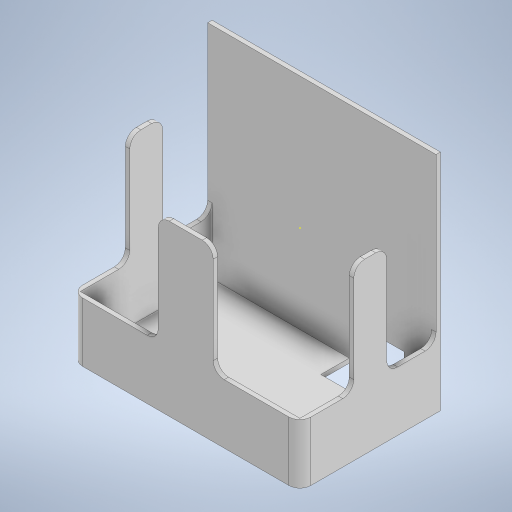
# Autodesk Inventor part: bag
Saved by Autodesk Inventor 2023 (Build 270158030, 158C)
## iProperties
Created: 2023-02-26
Part Number: bag
Material: Generic
Document SubType Name: Modeling
Designer: fatih
Density: 1 g/cm^3
Appearance: Default
Author: fatih
Autodesk Inventor part; units mm, degrees
ref_plane "YZ Plane" through (0, 0, 0) normal (1, 0, 0) x (0, 1, 0)
ref_plane "XZ Plane" through (0, 0, 0) normal (0, 1, 0) x (-1, 0, 0)
ref_plane "XY Plane" through (0, 0, 0) normal (0, 0, 1) x (1, 0, 0)
sketch "Sketch1" plane through (0, 0, 0) normal (0, 1, 0) x (-1, 0, 0)
  line L0 (0, 0) -> (0, -120)
  line L1 (0, 0) -> (200, 0)
  line L2 (200, 0) -> (200, -120)
  line L3 (200, -120) -> (0, -120)
  dimension "d0" = 120
  dimension "d1" = 200
  constraints: 8 end point, 2 perpendicular, 1 horizontal, 1 vertical
  measures "d0" distance of L0.start L0.end
  measures "d1" distance of L0.start L1.end
extrude "Extrusion1" add sketch "Sketch1" along normal blind 200
shell "Shell1" thickness 4 outward yes removed faces 1 at (-66.6667, 200, -40)
sketch "Sketch2" plane through (4, -4, 4) normal (1, 0, 0) x (0, 0, -1)
  line L0 (0, 0) -> (0, 204) projected
  line L1 (0, 0) -> (0, 204)
  line L2 (4, 4) -> (4, 104)
  line L3 (4, 4) -> (4, 204) projected
  line L4 (4, 54) -> (124, 54)
  line L5 (124, 4) -> (124, 204) projected
  line L6 (64, 54) -> (4, 54)
  line L7 (124, 54) -> (64, 54)
  line L8 (94, 54) -> (34, 54)
  line L9 (34, 54) -> (64, 54)
  line L10 (64, 54) -> (94, 54)
  line L11 (79, 54) -> (49, 54)
  line L12 (124, 104) -> (124, 204)
  line L13 (79, 154) -> (49, 154)
  line L14 (79, 54) -> (79, 154)
  line L15 (49, 54) -> (49, 154)
  line L16 (4, 54) -> (4, 204)
  line L17 (4, 204) -> (124, 204)
  line L18 (0, 204) -> (128, 204) projected
  line L19 (124, 204) -> (124, 54)
  constraints: 32 end point, 8 collinear, 8 midpoint, 4 perpendicular, 1 point on line, 1 vertical
extrude "Extrusion2" cut sketch "Sketch2" against normal through all contours L2 L3 L17 L5 L4 L14 L13 L15
sketch "Sketch3" plane through (-204, -4, 4) normal (0, 0, 1) x (1, 0, 0)
  line L0 (204, 54) -> (204, 154) projected
  line L1 (4, 4) -> (4, 54) projected
  line L2 (204, 54) -> (4, 54)
  line L3 (4, 54) -> (104, 54)
  line L4 (104, 54) -> (4, 54)
  line L5 (104, 54) -> (54, 54)
  line L6 (208, 54) -> (204, 54) projected
  line L7 (104, 54) -> (204, 54)
  line L8 (204, 54) -> (154, 54)
  line L9 (154, 54) -> (104, 54)
  line L10 (104, 54) -> (54, 54)
  line L11 (79, 54) -> (129, 54)
  line L12 (129, 154) -> (79, 154)
  line L13 (129, 54) -> (129, 154)
  line L14 (79, 54) -> (79, 154)
  line L15 (4, 54) -> (4, 204)
  line L16 (208, 204) -> (0, 204) projected
  line L17 (204, 54) -> (204, 204)
  line L18 (4, 54) -> (0, 54)
  line L19 (0, 0) -> (0, 204) projected
  line L20 (0, 204) -> (0, 54)
  line L21 (0, 204) -> (208, 204)
  line L22 (208, 154) -> (208, 54) projected
  line L23 (208, 0) -> (208, 204) projected
  line L24 (208, 54) -> (208, 204)
  line L25 (204, 54) -> (208, 54)
  point P0 (204, 4)
  constraints: 38 end point, 6 collinear, 5 midpoint, 4 horizontal, 3 perpendicular, 2 point on line, 2 vertical
extrude "Extrusion3" cut sketch "Sketch3" against normal blind 10 contours L2 L13 L12 L14 L15 L16 L17 L0 | L0 L17 L16 L23 L22 L6 | L15 L18 L19 L16
sketch "Sketch4" plane through (0, 200, 0) normal (0, 1, 0) x (1, 0, 0)
  point P0 (0, 0)
fillet "Fillet1" radius 10 16 edges at (2, 50, -45) (2, 50, -75) (2, 50, -120) (-75, 50, 2) (-125, 50, 2) (-202, 50, -45) (-202, 50, -75) (-202, 50, -120) (2, 150, -45) (2, 150, -75) (-75, 150, 2) (-125, 150, 2) (-202, 150, -45) (-202, 150, -75) (4, 23, 4) (-204, 23, 4)
sketch "Sketch5" plane through (4, -4, -124) normal (0, 0, -1) x (-1, 0, 0)
  line L0 (204, 4) -> (4, 4) projected
  line L1 (204, 4) -> (104, 4)
  line L2 (79, 4) -> (104, 4)
  line L3 (29, 4) -> (4, 4)
  line L4 (79, 4) -> (29, 4)
  line L5 (29, 4) -> (29, 34)
  line L6 (79, 4) -> (79, 34)
  line L7 (79, 34) -> (29, 34)
  line L8 (29, 4) -> (29, 0)
  line L9 (198, 0) -> (10, 0) projected
  line L10 (29, 0) -> (79, 0)
  line L11 (79, 0) -> (79, 4)
  line L12 (4, 4) -> (29, 4)
  line L13 (79, 4) -> (204, 4)
  line L14 (4, 4) -> (29, 4)
  line L15 (79, 4) -> (104, 4)
  dimension "d10" = 30
  constraints: 28 end point, 10 collinear, 3 perpendicular, 2 point on line, 2 vertical, 1 horizontal
  measures "d10" distance of L3.start L5.end
extrude "Extrusion4" cut sketch "Sketch5" against normal blind 10
sketch "Sketch6" plane through (0, -4, 0) normal (0, -1, 0) x (1, 0, 0)
  line L0 (-25, -114) -> (-25, -124) projected
  line L1 (-25, -124) -> (-25, -94)
  line L2 (-75, -124) -> (-75, -94)
  line L3 (-75, -94) -> (-25, -94)
  line L4 (-25, -124) -> (-75, -124) projected
  line L5 (-25, -124) -> (-75, -124)
  point P0 (0, 0)
  dimension "d13" = 30
  constraints: 8 end point, 2 equal length, 1 perpendicular, 1 vertical
  measures "d13" distance of L0.end L1.end
extrude "Extrusion5" cut sketch "Sketch6" against normal blind 10
body "Solid1"
